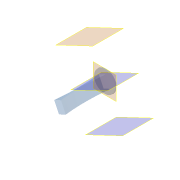
# Autodesk Inventor part: 00_lightshit_ray1
Saved by Autodesk Inventor 2019.4 (Build 234330000, 330)
## iProperties
Created: 2021-02-24
Part Number: 00_lightshit_ray1
Material: Generic
Document SubType Name: Modeling
Designer: diederichbenedict
Density: 1 g/cm^3
Appearance: Polycarbonate - Clear
Author: diederichbenedict
Autodesk Inventor part; units mm, degrees
ref_plane "YZ Plane" through (0, 0, 0) normal (1, 0, 0) x (0, 1, 0)
ref_plane "XZ Plane" through (0, 0, 0) normal (0, 1, 0) x (-1, 0, 0)
ref_plane "XY Plane" through (0, 0, 0) normal (0, 0, 1) x (1, 0, 0)
ref_plane "Work Plane3" through (-15.3296, -7.279, -15.06) normal (0.4289346, -0.9033355, 0) x (0.9033355, 0.4289346, 0)
ref_plane "Work Plane1" through (4.8151, 29.7955, -15.06) normal (-0.4289346, 0.9033355, 0) x (-0.9033355, -0.4289346, 0)
ref_plane "Work Plane2" through (-4.6706, -29.7269, -15.06) normal (0.4289346, -0.9033355, 0) x (0.9033355, 0.4289346, 0)
sketch "Sketch1" plane through (-15.3296, -7.279, -15.06) normal (0.4289346, -0.9033355, 0) x (0.9033355, 0.4289346, 0)
  circle A0 centre (16.97, 33.03) radius 7.5 projected
  line L0 (9.47, 15.06) -> (24.47, 15.06) projected
  arc A1 (20.0714, 51.4951) -> (20.0714, 15.06) centre (87.3367, 33.2775) ccw
  line L1 (20.0714, 15.06) -> (20.0714, 51.4951) construction
  line L2 (20.0714, 15.06) -> (56.5065, 15.06) construction
  line L3 (20.0714, 51.4951) -> (16.97, 51.4951)
  line L4 (16.97, 51.4951) -> (16.97, 15.06)
  line L5 (20.0714, 15.06) -> (16.97, 15.06)
  dimension "d0" = 90
  constraints: 10 end point, 2 horizontal, 2 perpendicular, 2 point on circle, 1 centre point, 1 collinear, 1 point on line
  measures "d0" angle of L2 L1
extrude "Extrusion1" add sketch "Sketch1" along normal mid plane 8 contours A1 A0 L4 | A0 L4 L3 A1 | A1 L0 L4 A0
ref_plane "Work Plane4" through (0, 0, 0) normal (0, 0, 1) x (1, 0, 0)
sketch "Sketch2" plane through (0, 0, 0) normal (0, 0, 1) x (1, 0, 0)
  circle A0 centre (0, 0) radius 7.5 projected
  point P0 (0, 0)
extrude "Extrusion2" add sketch "Sketch2" against normal blind 1
mirror "Mirror1" about plane through (0, 0, 36.4351) normal (-0.9033355, -0.4289346, 0) of "Extrusion1"
body "Solid1"
